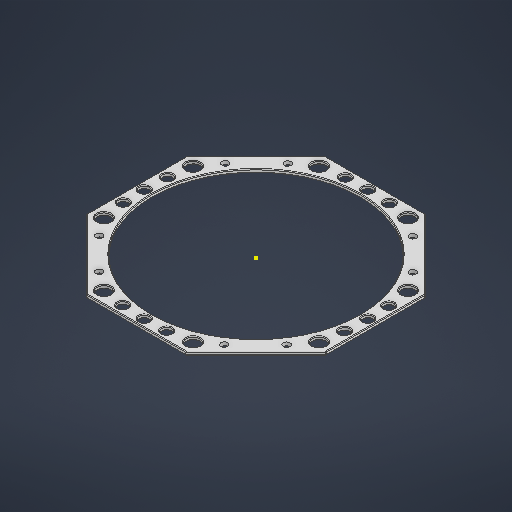
# Autodesk Inventor part: Part5
Saved by Autodesk Inventor 2026.2 (Build 302298000, 298)
## iProperties
Created: 2025-12-08
Part Number: Part5
Material: Generic
Document SubType Name: Modeling
Designer: Thoma
Density: 1 g/cm^3
Appearance: Default
Author: Thoma
Autodesk Inventor part; units mm, degrees
ref_plane "YZ Plane" through (0, 0, 0) normal (1, 0, 0) x (0, 1, 0)
ref_plane "XZ Plane" through (0, 0, 0) normal (0, 1, 0) x (-1, 0, 0)
ref_plane "XY Plane" through (0, 0, 0) normal (0, 0, 1) x (1, 0, 0)
sketch "Sketch1" plane through (0, 0, 0) normal (0, 1, 0) x (-1, 0, 0)
  line L0 (-72.4874, -175) -> (-175, -72.4874)
  line L1 (-175, -72.4874) -> (-175, 72.4874)
  line L2 (-175, 72.4874) -> (-72.4874, 175)
  line L3 (-72.4874, 175) -> (72.4874, 175)
  line L4 (72.4874, 175) -> (175, 72.4874)
  line L5 (175, 72.4874) -> (175, -72.4874)
  line L6 (175, -72.4874) -> (72.4874, -175)
  line L7 (72.4874, -175) -> (-72.4874, -175)
  circle A0 centre (0, 0) radius 152.4
  point P0 (0, 175)
  point P1 (0, -175)
  dimension "d0" = 350
  dimension "d1" = 304.8
  constraints: 16 end point, 2 coincident, 2 midpoint, 1 centre point, 17 other
  measures "d0" distance of point (0, 175) point (0, -175)
  measures "d1" diameter of A0
extrude "Extrusion1" add sketch "Sketch1" along normal blind 5
fillet "Fillet1" radius 1 20 edges at (-123.7437, 5, -123.7437) (-175, 5, 0) (-123.7437, 5, 123.7437) (0, 5, 175) (123.7437, 5, 123.7437) (175, 5, 0) (123.7437, 5, -123.7437) (0, 5, -175) (175, 0, 0) (175, 2.5, -72.4874) (175, 2.5, 72.4874) (-123.7437, 0, -123.7437) (0, 0, -175) (123.7437, 0, -123.7437) (123.7437, 0, 123.7437) (0, 0, 175) (-123.7437, 0, 123.7437) (-175, 0, 0) (152.4, 5, 0) (152.4, 0, 0)
sketch "Sketch2" plane through (0, 0, 0) normal (0, -1, 0) x (1, 0, 0)
  point P0 (0, 0)
sketch "Sketch3" plane through (0, 0, 0) normal (0, -1, 0) x (1, 0, 0)
  line L0 (174, 72.0732) -> (72.0732, 174) projected
  circle A0 centre (0, 0) radius 152.4 projected
  line L1 (174, -72.0732) -> (174, 72.0732) projected
  circle A1 centre (157.3996, 65.1971) radius 10
  dimension "d5" = 20
  constraints: 1 centre point
  measures "d5" diameter of A1
extrude "Extrusion2" cut sketch "Sketch3" against normal blind 5 contours A1
pattern_circular "Circular Pattern1" count 8 over 360 about axis through (0, -10, 0) along (0, 1, 0) of "Extrusion2"
fillet "Fillet2" radius 1 2 edges at (58.126, 5, 150.3286) (58.126, 0, 150.3286)
pattern_circular "Circular Pattern2" count 8 over 360 about axis through (0, -10, 0) along (0, 1, 0) of "Fillet2"
sketch "Sketch5" plane through (0, 5, 0) normal (0, 1, 0) x (1, 0, 0)
  line L0 (175, -72.0732) -> (174, -72.0732) projected
  line L1 (174, -72.0732) -> (141.7231, -58.7036)
  circle A0 centre (0, 0) radius 153.4 projected
  line L2 (174, 72.0732) -> (141.7231, 58.7036)
  circle A1 centre (157.3996, 65.1971) radius 11 projected
  circle A2 centre (162.2989, -32.8297) radius 7.5
  circle A3 centre (163.7, 0) radius 7.5
  circle A4 centre (162.508, 31.7784) radius 7.5
  circle A5 centre (32.8297, 162.2989) radius 7.5
  circle A6 centre (0, 163.7) radius 7.5
  circle A7 centre (-31.7784, 162.508) radius 7.5
  circle A8 centre (-162.2989, 32.8297) radius 7.5
  circle A9 centre (-163.7, 0) radius 7.5
  circle A10 centre (-162.508, -31.7784) radius 7.5
  circle A11 centre (-32.8297, -162.2989) radius 7.5
  circle A12 centre (0, -163.7) radius 7.5
  circle A13 centre (31.7784, -162.508) radius 7.5
  dimension "d22" = 45
  dimension "d24" = 15
  dimension "d25" = 15
  dimension "d28" = 22.5
  dimension "d32" = 360
  constraints: 12 centre point, 4 end point, 1 coincident, 35 other
  measures "d24" diameter of A2
  measures "d25" diameter of A3
extrude "Extrusion3" cut sketch "Sketch5" against normal blind 5 contours A2 | A3 | A4
pattern_circular "Circular Pattern3" count 4 over 360 about axis through (0, -10, 0) along (0, 1, 0) of "Extrusion3"
fillet "Fillet3" radius 1 6 edges at (-155.008, 5, 31.7784) (-155.008, 0, 31.7784) (-156.2, 0, 0) (-154.7989, 0, -32.8297) (-156.2, 5, 0) (-154.7989, 5, -32.8297)
pattern_circular "Circular Pattern4" count 4 over 360 about axis through (0, -10, 0) along (0, 1, 0) of "Fillet3"
sketch "Sketch7" plane through (0, 5, 0) normal (0, 1, 0) x (1, 0, 0)
  line L0 (174, -72.0732) -> (72.0732, -174) projected
  line L1 (72.0732, -174) -> (58.7036, -141.7231)
  circle A0 centre (0, 0) radius 153.4 projected
  line L2 (174, -72.0732) -> (141.7231, -58.7036)
  circle A1 centre (163.7, 0) radius 8.5 projected
  circle A2 centre (163.7, 0) radius 7.5 projected
  line L3 (171.2, 0) -> (156.2, 0)
  line L4 (121.0567, -121.0567) -> (110.4501, -110.4501)
  arc A3 (65.3884, -157.8616) -> (87.6514, -141.1105) centre (-145.2272, 145.2272) ccw
  circle A4 centre (91.509, -137.9295) radius 5
  circle A5 centre (137.3266, -92.4113) radius 5
  arc A6 (95.3231, -134.6965) -> (115.7534, -115.7534) centre (-145.2272, 145.2272) ccw
  arc A7 (115.7534, -115.7534) -> (133.9937, -96.1385) centre (-145.2272, 145.2272) ccw
  arc A8 (140.4274, -88.4889) -> (157.8616, -65.3884) centre (-145.2272, 145.2272) ccw
  dimension "d45" = 45
  dimension "d47" = 10
  dimension "d50" = 22.5
  constraints: 16 point on circle, 8 end point, 6 centre point, 4 midpoint, 2 line through centre, 1 horizontal, 7 other
  measures "d47" diameter of A4
extrude "Extrusion4" cut sketch "Sketch7" against normal blind 5 contours A5 | A4
pattern_circular "Circular Pattern5" count 4 over 360 about axis through (0, -10, 0) along (0, 1, 0) of "Extrusion4"
body "Solid1"
